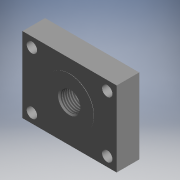
# Autodesk Inventor part: 36126 KSZ-M12x1,25
Saved by Autodesk Inventor 2017.3 (Build 213256000, 256)
## iProperties
Part Number: 36126 KSZ-M12x1,25
Material: Generic
Catalog Web Link: www.cadenas.de
Description: KSZ-coupling piece
Vendor: FESTO
Document SubType Name: Modeling
Designer: partserver
Manufacturer: FESTO
Mass: 180 g
Surface Area: 78.6432 cm^2
Volume: 23.1053 cm^3
Density: 1 g/cm^3
Appearance: PSOLRGB-175-175-175
Category: PARTsolutions
Company: FESTO
Title: 36126 KSZ-M12x1,25
Author: Cadenas PARTsolutions
Comments: coupling piece
PSOL_IDENT_0: {$CADENAS_DATA\23d-libs\festo\parts\k\ksz\ksz.prj},173 {VTYP=3D},{NB=36126 KSZ-M12x1,25},{LINA=36126
PSOL_IDENT_1: KSZ-M12x1,25},{NN=KSZ},{DATE=20.03.2020 14:05:39},{GEOMDATE=19.03.2020 13:58:18},{VERSION=},{LINEID=
PSOL_IDENT_2: 40},{WBVAR=},{WBNUMERIC=}  {NB=36126 KSZ-M12x1,25},{LINA=36126 KSZ-M12x1,25},{KT=DUMMY},{TNR=36126},
PSOL_IDENT_3: {TYP=KSZ-M12x1,25},{B1=50.000},{B2=40.000},{B3=40.000},{B4=30.000},{D1=17.000},{D2=26.000},{D3=5.500
PSOL_IDENT_4: },{H1=22.000},{H2=12.000},{KK=M12x1.25},{KKNDR=12.000},{KKP=1.250},{T1=5.950},{T=0.000},{SW1=15.000}
PSOL_IDENT_5: ,{Z=0.000},{INCH=0},{CNSMASSEXACT=0.180}
NB: 36126 KSZ-M12x1,25
NN: KSZ
NT: coupling piece
NBSYN: $TNR. $TYP.
LINA: 36126 KSZ-M12x1,25
CATALOG: Festo
TNR: 36126
TYP: KSZ-M12x1,25
B1: 50
B2: 40
B3: 40
B4: 30
D1: 17
D2: 26
D3: 5.5
H1: 22
H2: 12
KK: M12x1.25
T1: 5.95
T: 0
SW1: 15
Z: 0
CNSMASSEXACT: 0.18
SUPPLIER: FESTO
ARTICLENO: 36126 KSZ-M12x1,25
BOMINFO: 36126 KSZ-M12x1,25
CREATOR: CADENAS GmbH
Autodesk Inventor part; units mm, degrees
sketch "Skizze_1" plane through (0, 0, 0) normal (0, 1, 0) x (-1, 0, 0)
  line L0 (25, 20) -> (-25, 20)
  line L1 (-25, 20) -> (-25, -20)
  line L2 (-25, -20) -> (25, -20)
  line L3 (25, -20) -> (25, 20)
  circle A0 centre (-20, -15) radius 2.75
  circle A1 centre (-20, 15) radius 2.75
  circle A2 centre (20, -15) radius 2.75
  circle A3 centre (20, 15) radius 2.75
  constraints: 8 end point, 4 centre point
extrude "Extrusion1" add sketch "Skizze_1" along normal blind 12
sketch "Skizze_2" plane through (0, 0, 0) normal (0, 0, 1) x (1, 0, 0)
  line L0 (0, -0.15) -> (0, 21.85)
  line L1 (0, 21.85) -> (8.5, 21.85)
  line L2 (8.5, 21.85) -> (8.5, 5.8)
  line L3 (8.5, 5.8) -> (13, 5.8)
  line L4 (13, 5.8) -> (13, -0.15)
  line L5 (13, -0.15) -> (0, -0.15)
  line L6 (0, -0.15) -> (0, 21.85)
  constraints: 14 end point
revolve "Revolution1" add sketch "Skizze_2" angle 360 about axis through (0, -0.15, 0) along (0, -1, 0)
sketch "Skizze_3" plane through (0, 21.85, 0) normal (0, 1, 0) x (1, 0, 0)
  line L0 (-15, -15) -> (15, -15)
  line L1 (15, -15) -> (15, -7.5)
  line L2 (15, -7.5) -> (-13.5, -7.5)
  line L3 (-13.5, -7.5) -> (-13.5, 7.5)
  line L4 (-13.5, 7.5) -> (15, 7.5)
  line L5 (15, 7.5) -> (15, 15)
  line L6 (15, 15) -> (-15, 15)
  line L7 (-15, 15) -> (-15, -15)
  constraints: 16 end point
extrude "Extrusion2" cut sketch "Skizze_3" along normal mid plane 17.6
sketch "Skizze_6" plane through (0, 0, 0) normal (0, 0, 1) x (1, 0, 0)
  line L0 (0, -0.15) -> (0, 21.85)
  line L1 (0, 21.85) -> (6, 21.85)
  line L2 (6, 21.85) -> (5.3235, 21.1735)
  line L3 (5.3235, 21.1735) -> (5.3235, 0.5265)
  line L4 (5.3235, 0.5265) -> (6, -0.15)
  line L5 (6, -0.15) -> (0, -0.15)
  line L6 (0, -0.15) -> (0, 21.85)
  constraints: 14 end point
revolve "Revolution2" cut sketch "Skizze_6" angle 360 about axis through (0, -0.15, 0) along (0, -1, 0)
thread "Thread1" size "M12x1.25" class "6H" standard "ISO Metric profile" full length
ref_plane "FDT_CYLINDER_XY" through (0, 22, 0) normal (0, 1, 0) x (1, 0, 0)
ref_plane "FDT_CYLINDER_YZ" through (0, 22, 0) normal (1, 0, 0) x (0, 0, -1)
ref_plane "FDT_CYLINDER_ZX" through (0, 22, 0) normal (0, 0, -1) x (0, 1, 0)
body "Solid1"
